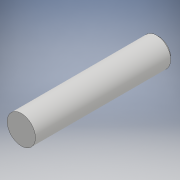
# Autodesk Inventor part: parte1_cilindro
Saved by Autodesk Inventor 2018 (Build 220112000, 112)
## iProperties
Created: 2018-04-06
Part Number: parte1_cilindro
Material: Generic
Document SubType Name: Modeling
Designer: Francisco
Density: 1 g/cm^3
Appearance: Default
Author: Francisco
Autodesk Inventor part; units mm, degrees
ref_plane "YZ Plane" through (0, 0, 0) normal (1, 0, 0) x (0, 1, 0)
ref_plane "XZ Plane" through (0, 0, 0) normal (0, 1, 0) x (-1, 0, 0)
ref_plane "XY Plane" through (0, 0, 0) normal (0, 0, 1) x (1, 0, 0)
sketch "Sketch1" plane through (0, 0, 0) normal (0, 0, 1) x (1, 0, 0)
  line L0 (-7, -27.989) -> (-7, 39.011)
  line L1 (-7, 39.011) -> (-5.9393, 40.0716)
  line L2 (-7, 39.011) -> (-5.5, 39.011) construction
  line L3 (-5.9393, 40.0716) -> (-4.1012, 40.0716)
  line L4 (0, 40.7587) -> (0, -33.1319) construction
  line L5 (-4.1012, 40.0716) -> (0, 40.0716)
  line L6 (-7, -27.989) -> (0, -27.989)
  line L7 (0, -27.989) -> (0, 40.0716)
  point P0 (0, 0)
  dimension "d0" = 67
  dimension "d1" = 1.5
  dimension "d2" = 45
  dimension "d3" = 14
  constraints: 16 end point, 3 horizontal, 3 point on line, 2 vertical, 1 collinear, 1 equal length, 1 perpendicular
  measures "d0" distance of L0.start L0.end
  measures "d1" distance of L0.end L1.end
  measures "d2" angle of L2 L1
  measures "d3" diameter of L0 L4
revolve "Revolution1" add sketch "Sketch1" angle 360 about axis through (0, 40.7587, 0) along (0, -1, 0)
body "Solid1"
